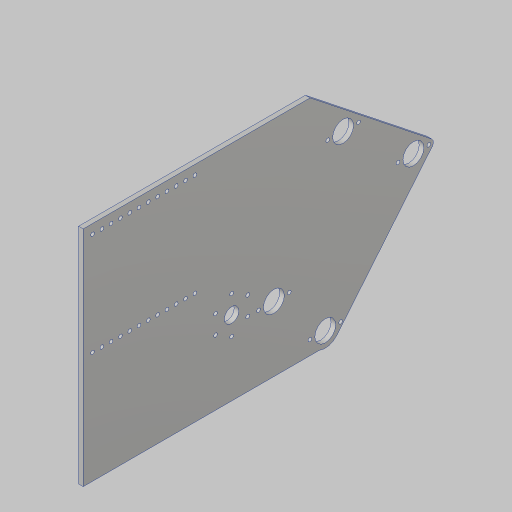
# Autodesk Inventor part: GI - 001
Saved by Autodesk Inventor 2023.5 (Build 275446000, 446)
## iProperties
Created: 2025-01-17
Part Number: GI - 001
Material: Aluminum 6061
Document SubType Name: Modeling
Designer: mavericks
Density: 2.7 g/cm^3
Appearance: Aluminum - Flat
Mass: 1813.75 g
Surface Area: 2253.74 cm^2
Volume: 671.761 cm^3
Author: mavericks
Autodesk Inventor part; units mm, degrees
ref_plane "YZ Plane" through (0, 0, 0) normal (1, 0, 0) x (0, 1, 0)
ref_plane "XZ Plane" through (0, 0, 0) normal (0, 1, 0) x (-1, 0, 0)
ref_plane "XY Plane" through (0, 0, 0) normal (0, 0, 1) x (1, 0, 0)
sketch "Sketch2" plane through (0, 0, 0) normal (1, 0, 0) x (0, 1, 0)
  line L0 (63.5, 38.1) -> (-63.5, 38.1) construction
  line L1 (-63.5, 38.1) -> (-63.5, -38.1) construction
  line L2 (-63.5, -38.1) -> (63.5, -38.1) construction
  line L3 (63.5, -38.1) -> (63.5, 38.1) construction
  line L4 (63.5, 38.1) -> (-63.5, -38.1) construction
  line L5 (-63.5, 38.1) -> (63.5, -38.1) construction
  line L6 (-63.5, 38.1) -> (-76.2, 38.1) construction
  line L7 (-76.2, 38.1) -> (-76.2, -266.7) construction
  line L8 (-76.2, -266.7) -> (-63.5, -266.7) construction
  line L9 (-63.5, -266.7) -> (-63.5, 38.1) construction
  circle A0 centre (-25.8145, -515.3533) radius 57.15 construction
  circle A1 centre (-50.8, -140.0055) radius 15.875 construction
  circle A2 centre (19.05, -69.85) radius 25.4 construction
  circle A3 centre (98.425, -260.3407) radius 63.5 construction
  circle A4 centre (98.425, -260.3407) radius 14.2875
  circle A5 centre (172.9213, -164.3575) radius 63.5 construction
  circle A6 centre (172.9213, -164.3575) radius 14.2875
  circle A7 centre (-50.8, -140.0055) radius 14.2875
  circle A8 centre (19.05, -69.85) radius 14.2875
  line L10 (-69.85, 38.1) -> (-69.85, -147.943)
  line L11 (-57.15, 38.1) -> (-6.35, 38.1) construction
  line L12 (-6.35, 38.1) -> (-6.35, 444.5) construction
  line L13 (-6.35, 444.5) -> (-57.15, 444.5) construction
  line L14 (-57.15, 444.5) -> (-57.15, 38.1) construction
  line L15 (172.9213, -185.376) -> (172.9213, -143.339) construction
  line L16 (98.425, -239.3222) -> (98.425, -281.3592) construction
  line L17 (19.05, -48.8315) -> (19.05, -90.8685) construction
  line L18 (-50.8, -118.987) -> (-50.8, -161.024) construction
  circle A9 centre (98.425, -281.3592) radius 6.35 construction
  circle A10 centre (98.425, -260.3407) radius 20.6375 construction
  circle A11 centre (172.9213, -164.3575) radius 20.6375 construction
  circle A12 centre (-50.8, -140.0055) radius 20.6375 construction
  line L19 (234.95, -119.3167) -> (103.4016, -285.3033)
  line L20 (-63.9166, -155.9384) -> (94.3891, -286.2616)
  arc A13 (-69.85, -132.068) -> (-63.9166, -155.9384) centre (-50.8, -140.0055) ccw
  arc A14 (94.3891, -286.2616) -> (103.4016, -285.3033) centre (98.425, -281.3592) ccw
  line L21 (-69.85, 38.1) -> (-69.85, 190.5)
  line L22 (-69.85, 190.5) -> (234.95, 190.5)
  line L23 (234.95, 190.5) -> (234.95, -119.3167)
  line L24 (199.0311, -58.2205) -> (108.7364, 11.8607)
  line L25 (108.7364, 11.8607) -> (-76.2, -226.4168)
  line L26 (-76.2, -226.4168) -> (14.0946, -296.4979)
  line L27 (14.0946, -296.4979) -> (199.0311, -58.2205)
  circle A15 centre (172.9213, -164.3575) radius 44.45 construction
  circle A16 centre (98.425, -260.3407) radius 44.45 construction
  line L28 (63.5, 38.1) -> (63.5, 190.5) construction
  line L29 (152.4, 38.1) -> (152.4, 190.5) construction
  line L30 (222.25, 114.3) -> (82.55, 114.3) construction
  point P0 (0, 0)
  point P1 (-14.3002, 165.1)
  point P2 (-49.1998, 165.1)
  point P3 (-14.3002, 190.5)
  point P4 (-49.1998, 190.5)
  point P5 (-14.3002, 215.9)
  point P6 (-49.1998, 215.9)
  point P7 (-14.3002, 241.3)
  point P8 (-49.1998, 241.3)
  point P9 (-31.75, 38.1)
  point P10 (222.25, 177.8)
  point P11 (222.25, 165.1)
  point P12 (222.25, 152.4)
  point P13 (222.25, 139.7)
  point P14 (222.25, 127)
  point P15 (222.25, 101.6)
  point P16 (222.25, 88.9)
  point P17 (222.25, 76.2)
  point P18 (222.25, 63.5)
  point P19 (222.25, 50.8)
  point P20 (222.25, 38.1)
  point P21 (63.5, 114.3)
  point P22 (152.4, 114.3)
  point P23 (152.4, 114.3)
  point P24 (152.4, 114.3)
  point P25 (82.55, 177.8)
  point P26 (82.55, 165.1)
  point P27 (82.55, 152.4)
  point P28 (82.55, 139.7)
  point P29 (82.55, 127)
  point P30 (82.55, 101.6)
  point P31 (82.55, 88.9)
  point P32 (82.55, 76.2)
  point P33 (82.55, 63.5)
  point P34 (82.55, 50.8)
  point P35 (82.55, 38.1)
  dimension "d2" = 127
  dimension "d3" = 76.2
  dimension "d4" = 12.7
  dimension "d5" = 304.8
  dimension "d6" = 114.3
  dimension "d7" = 31.75
  dimension "d8" = 50.8
  dimension "d9" = 127
  dimension "d10" = 174.625
  dimension "d11" = 28.575
  dimension "d12" = 31.75
  dimension "d13" = 25.4
  dimension "d14" = 98.999
  dimension "d16" = 222.2407
  dimension "d17" = 127
  dimension "d18" = 121.5009
  dimension "d20" = 28.575
  dimension "d21" = 28.575
  dimension "d22" = 28.575
  dimension "d40" = 50.8
  dimension "d41" = 19.05
  dimension "d42" = 406.4
  dimension "d43" = 127
  dimension "d44" = 7.9502
  dimension "d45" = 7.9502
  dimension "d48" = 25.4
  dimension "d70" = 180.577
  dimension "d80" = 42.037
  dimension "d81" = 42.037
  dimension "d82" = 42.037
  dimension "d83" = 42.037
  dimension "d84" = 12.7
  dimension "d85" = 6.35
  dimension "d86" = 6.35
  dimension "d87" = 6.35
  dimension "d97" = 152.4
  dimension "d98" = 12.7
  dimension "d101" = 12.7
  dimension "d104" = 12.7
  dimension "d109" = 114.3
  dimension "d110" = 301.625
  dimension "d111" = 19.05
  dimension "d112" = 95.25
  dimension "d113" = 304.8
  dimension "d114" = 139.7
  constraints: 62 end point, 17 centre point, 13 coincident, 11 midpoint, 11 symmetric about line, 9 point on circle, 8 parallel, 8 perpendicular, 8 vertical, 6 tangent, 5 point on line, 4 horizontal, 2 horizontal alignment, 1 equal radius, 1 vertical alignment, 17 other
  measures "d2" distance of L2.end L1.end
  measures "d3" distance of L1.end L0.end
  measures "d4" distance of L8.end L7.end
  measures "d5" distance of L7.end L6.end
  measures "d6" diameter of A0
  measures "d7" diameter of A1
  measures "d8" diameter of A2
  measures "d9" diameter of A3
  measures "d10" distance from line of A3.centre L7
  measures "d11" diameter of A4
  measures "d12" distance from line of A2.centre L2
  measures "d13" distance from line of L7 A1.centre
  measures "d14" distance of A2.centre A1.centre
  measures "d16" distance from line of L2 A3.centre
  measures "d17" diameter of A5
  measures "d18" distance of A3.centre A5.centre
  measures "d20" diameter of A6
  measures "d21" diameter of A7
  measures "d22" diameter of A8
  measures "d40" distance of L13.end L12.end
  measures "d41" distance between parallel lines of L14 L7
  measures "d42" distance of L13.end L11.start
  measures "d43" distance from line of L0 point (-14.3, 165.1)
  measures "d44" distance from line of L12 point (-14.3, 165.1)
  measures "d45" distance from line of L14 point (-49.2, 165.1)
  measures "d48" distance of point (-14.3, 165.1) point (-14.3, 190.5)
  measures "d70" distance of A2.centre A5.centre
  measures "d80" distance of L15.start L15.end
  measures "d81" distance of L16.start L16.end
  measures "d82" distance of L17.start L17.end
  measures "d83" distance of L18.start L18.end
  measures "d84" diameter of A9
  measures "d85" radial gap between concentric circles of A4 A10
  measures "d86" radial gap between concentric circles of A6 A11
  measures "d87" radial gap between concentric circles of A7 A12
  measures "d97" distance between parallel lines of L0 L22
  measures "d98" distance from line of L23 point (222.25, 177.8)
  measures "d101" distance from line of L22 point (222.25, 177.8)
  measures "d104" distance of point (222.25, 177.8) point (222.25, 165.1)
  measures "d109" distance of L26.end L25.end
  measures "d110" distance of L25.end L24.end
  measures "d111" radial gap between concentric circles of A5 A15
  measures "d112" distance from line of L7 A2.centre
  measures "d113" distance of L21.end L22.end
  measures "d114" distance of L30.start L30.end
extrude "Extrusion1" add sketch "Sketch2" along normal blind 6.35 contours L21 L22 L23 L19 A14 L20 L27 L24 L25 A13 L10 | L10 A13 | L25 L24 L27 L20
sketch "Sketch3" plane through (6.35, 0, 0) normal (1, 0, 0) x (0, 0, -1)
  line L0 (-38.1, 63.5) -> (38.1, 63.5) construction
  line L1 (38.1, 63.5) -> (38.1, -63.5) construction
  line L2 (38.1, -63.5) -> (-38.1, -63.5) construction
  line L3 (-38.1, -63.5) -> (-38.1, 63.5) construction
  line L4 (-38.1, 63.5) -> (38.1, -63.5) construction
  line L5 (38.1, 63.5) -> (-38.1, -63.5) construction
  line L6 (-190.5, -69.85) -> (132.068, -69.85) construction
  point P0 (0, 0)
  point P1 (0, 0)
  point P2 (147.943, -69.85)
  dimension "d36" = 76.2
  dimension "d37" = 127
  dimension "d38" = 6.35
  constraints: 12 end point, 2 midpoint, 2 parallel, 1 horizontal, 1 perpendicular
  measures "d36" distance of L1.end L2.end
  measures "d37" distance of L0.end L1.end
  measures "d38" distance between parallel lines of L6 L2
sketch "Sketch4" plane through (0, 0, 0) normal (-1, 0, 0) x (0, 0, 1)
  circle A0 centre (-12.1007, 31.75) radius 9.906
  line L0 (190.5, -69.85) -> (-132.068, -69.85) projected
  line L1 (190.5, -69.85) -> (-132.068, -69.85) projected
  circle A1 centre (-12.1007, 31.75) radius 25.4 construction
  circle A2 centre (-69.85, 19.05) radius 14.2875 projected
  circle A3 centre (-140.0055, -50.8) radius 14.2875 projected
  circle A4 centre (-164.3575, 172.9213) radius 14.2875 projected
  circle A5 centre (-260.3407, 98.425) radius 14.2875 projected
  arc A6 (-155.9384, -63.9166) -> (-132.068, -69.85) centre (-140.0055, -50.8) ccw projected
  line L2 (-155.9384, -63.9166) -> (-286.2616, 94.3891) projected
  arc A7 (-285.3033, 103.4016) -> (-286.2616, 94.3891) centre (-281.3592, 98.425) ccw projected
  line L3 (-285.3033, 103.4016) -> (-119.3167, 234.95) projected
  line L4 (-119.3167, 234.95) -> (190.5, 234.95) projected
  line L5 (190.5, 234.95) -> (190.5, -69.85) projected
  circle A8 centre (-69.85, 19.05) radius 14.2875 projected
  circle A9 centre (-140.0055, -50.8) radius 14.2875 projected
  circle A10 centre (-164.3575, 172.9213) radius 14.2875 projected
  circle A11 centre (-260.3407, 98.425) radius 14.2875 projected
  arc A12 (-155.9384, -63.9166) -> (-132.068, -69.85) centre (-140.0055, -50.8) ccw projected
  line L6 (-155.9384, -63.9166) -> (-286.2616, 94.3891) projected
  arc A13 (-285.3033, 103.4016) -> (-286.2616, 94.3891) centre (-281.3592, 98.425) ccw projected
  line L7 (-285.3033, 103.4016) -> (-119.3167, 234.95) projected
  line L8 (-119.3167, 234.95) -> (190.5, 234.95) projected
  line L9 (190.5, 234.95) -> (190.5, -69.85) projected
  point P0 (0, 0)
  point P1 (-69.85, -12.7)
  point P2 (-12.1007, 57.15)
  point P3 (-34.0977, 44.45)
  point P4 (-34.0977, 19.05)
  point P5 (-12.1007, 6.35)
  point P6 (9.8964, 19.05)
  point P7 (9.8964, 44.45)
  dimension "d58" = 50.8
  dimension "d53" = 19.812
  dimension "d54" = 72.8751
  dimension "d55" = 101.6
  dimension "d61" = 360
  constraints: 2 vertical alignment, 1 centre point, 1 coincident, 9 other
  measures "d53" diameter of A0
  measures "d54" distance of A0.centre point (-69.85, -12.7)
  measures "d55" distance from line of L0 A0.centre
extrude "Extrusion2" cut sketch "Sketch4" against normal blind 25.4 contours A0
hole "Hole1" at (0, 57.15, -12.1007) at (0, 44.45, -34.0977) at (0, 19.05, -34.0977) at (0, 6.35, -12.1007) at (0, 19.05, 9.8964) at (0, 44.45, 9.8964) direction (1, 0, 0) diameter 5.1054 end through all clearance for "Flat Head Machine Screw (82)" size "#10" standard "Ansi Unified Screw Threads"
hole "Hole3" at (0, -14.3002, 215.9) at (0, -49.1998, 215.9) at (0, -14.3002, 241.3) at (0, -49.1998, 241.3) at (0, 172.9213, -185.376) at (0, 172.9213, -143.339) at (0, 98.425, -239.3222) at (0, 98.425, -281.3592) at (0, 19.05, -48.8315) at (0, 19.05, -90.8685) at (0, -50.8, -118.987) at (0, -50.8, -161.024) at (0, 222.25, 177.8) at (0, 222.25, 165.1) at (0, 222.25, 152.4) at (0, 222.25, 139.7) at (0, 222.25, 127) at (0, 222.25, 114.3) at (0, 222.25, 101.6) at (0, 222.25, 88.9) at (0, 222.25, 76.2) at (0, 222.25, 63.5) at (0, 222.25, 50.8) at (0, 222.25, 38.1) at (0, 82.55, 38.1) at (0, 82.55, 50.8) at (0, 82.55, 63.5) at (0, 82.55, 76.2) at (0, 82.55, 88.9) at (0, 82.55, 101.6) at (0, 82.55, 114.3) at (0, 82.55, 127) at (0, 82.55, 139.7) at (0, 82.55, 152.4) at (0, 82.55, 165.1) at (0, 82.55, 177.8) direction (1, 0, 0) diameter 5.1054 end through all clearance for "Flat Head Machine Screw (82)" size "#10" standard "Ansi Unified Screw Threads"
sketch "Sketch6" plane through (6.35, 0, 0) normal (1, 0, 0) x (0, 0, -1)
  line L0 (-190.5, -69.85) -> (132.068, -69.85) projected
  line L1 (-190.5, -69.85) -> (-38.1, -69.85)
  line L2 (-38.1, -69.85) -> (-38.1, 57.15)
  line L3 (-38.1, 57.15) -> (-190.5, 57.15)
  line L4 (-190.5, 57.15) -> (-190.5, -69.85)
  point P0 (0, 0)
  dimension "d115" = 127
  dimension "d116" = 152.4
  constraints: 8 end point, 2 parallel, 1 horizontal, 1 perpendicular
  measures "d115" distance between parallel lines of L0 L3
  measures "d116" distance between parallel lines of L4 L2
body "Solid1"
